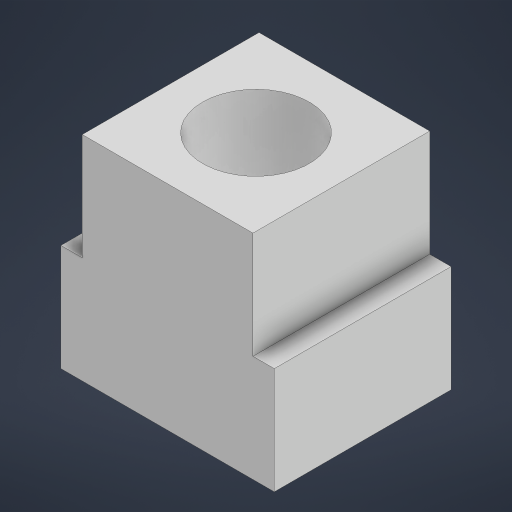
# Autodesk Inventor part: Part1
Saved by Autodesk Inventor 2024.3 (Build 283343000, 343)
## iProperties
Created: 2025-07-04
Part Number: Part1
Material: Generic
Document SubType Name: Modeling
Designer: LeoFB
Density: 1 g/cm^3
Appearance: Default
Author: LeoFB
Autodesk Inventor part; units mm, degrees
ref_plane "YZ Plane" through (0, 0, 0) normal (1, 0, 0) x (0, 1, 0)
ref_plane "XZ Plane" through (0, 0, 0) normal (0, 1, 0) x (-1, 0, 0)
ref_plane "XY Plane" through (0, 0, 0) normal (0, 0, 1) x (1, 0, 0)
sketch "Sketch2" plane through (0, 0, 0) normal (0, 1, 0) x (-1, 0, 0)
  line L0 (-5, 5) -> (5, 5)
  line L1 (5, 5) -> (5, -5)
  line L2 (5, -5) -> (-5, -5)
  line L3 (-5, -5) -> (-5, 5)
  line L4 (-5, 5) -> (5, -5) construction
  line L5 (5, 5) -> (-5, -5) construction
  circle A0 centre (0, 0) radius 2.5
  line L6 (5, 4.1414) -> (-5, 4.1414)
  line L7 (-5, -4.1414) -> (5, -4.1414)
  point P0 (5, -4.1414)
  dimension "d0" = 10
  dimension "d1" = 10
  dimension "d2" = 5
  dimension "d5" = 180
  constraints: 16 end point, 2 midpoint, 2 parallel, 2 perpendicular, 2 point on line, 1 centre point, 1 coincident, 1 horizontal, 4 other
  measures "d0" distance of L1.end L2.end
  measures "d1" distance of L0.end L1.end
  measures "d2" diameter of A0
extrude "Extrusion1" add sketch "Sketch2" along normal blind 10 contours L6 L1 L7 L3
sketch "Sketch3" plane through (0, 10, 0) normal (0, 1, 0) x (1, 0, 0)
  line L0 (5, 4.1414) -> (-5, 4.1414) projected
  line L1 (-5, -4.1414) -> (5, -4.1414) projected
  line L2 (-5, 4.1414) -> (-4, 4.1414)
  line L3 (-4, 4.1414) -> (-4, -4.1414)
  line L4 (-4, -4.1414) -> (-5, -4.1414)
  line L5 (-5, -4.1414) -> (-5, 4.1414)
  line L6 (5, -4.1414) -> (4, -4.1414)
  line L7 (4, -4.1414) -> (4, 4.1414)
  line L8 (4, 4.1414) -> (5, 4.1414)
  line L9 (5, 4.1414) -> (5, -4.1414)
  point P0 (0, 0)
  dimension "d9" = 1
  dimension "d12" = 180
  constraints: 16 end point, 2 parallel, 1 horizontal, 1 perpendicular, 1 point on line, 10 other
  measures "d9" distance of L3.end L4.end
extrude "Extrusion2" cut sketch "Sketch3" against normal blind 5 contours L9 L1 L7 L0 | L3 L1 L5 L0
body "Solid1"
